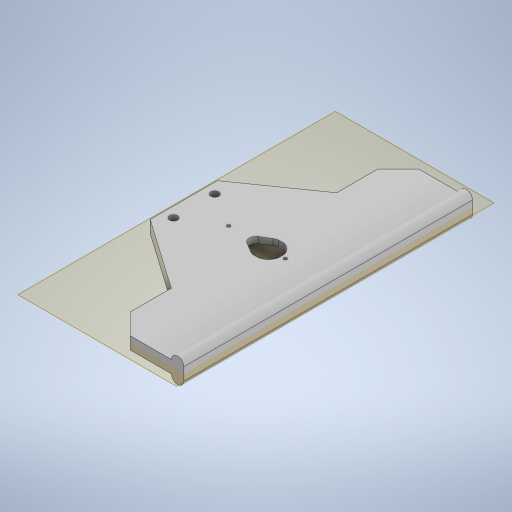
# Autodesk Inventor part: gripper_head 1
Saved by Autodesk Inventor 2023 (Build 270158000, 158)
## iProperties
Created: 2024-07-03
Part Number: gripper_head 1
Material: Generic
Document SubType Name: Modeling
Designer: Swoby
Density: 1 g/cm^3
Appearance: Default
Author: Swoby
Autodesk Inventor part; units mm, degrees
ref_plane "YZ Plane" through (0, 0, 0) normal (1, 0, 0) x (0, 1, 0)
ref_plane "XY Plane" through (0, 0, 0) normal (0, 0, 1) x (1, 0, 0)
sketch "Sketch1" plane through (0, 0, 0) normal (0, 0, 1) x (1, 0, 0)
  line L0 (-67, 3) -> (-67, -3)
  line L1 (-67, -3) -> (-3, -3)
  line L2 (-67, 3) -> (-3, 3)
  line L3 (0, -3) -> (0, 3) construction
  line L4 (3, -3) -> (3, 3)
  line L5 (-3, 3) -> (-3, -3)
  arc A0 (-3, -3) -> (3, -3) centre (0, -3) ccw
  arc A1 (3, 3) -> (-3, 3) centre (0, 3) ccw
  point P0 (0, 0)
  point P1 (-3, -3)
  dimension "d0" = 70
  dimension "d1" = 3
  dimension "d2" = 6
  dimension "d3" = 6
  constraints: 14 end point, 4 point on circle, 4 tangent, 2 centre point, 1 midpoint, 1 parallel, 1 perpendicular, 1 point on line, 1 vertical
  measures "d0" distance between parallel lines of L4 L0
  measures "d1" radius of A1
  measures "d2" distance between parallel lines of L1 L2
  measures "d3" distance of L3.start L3.end
extrude "Extrusion1" add sketch "Sketch1" along normal mid plane 140
sketch "Sketch2" plane through (-67, 3, 70) normal (0, 1, 0) x (1, 0, 0)
  line L0 (0, 0) -> (64, 0) projected
  line L1 (64, 0) -> (44, 0)
  line L2 (0, 140) -> (0, 0) projected
  line L3 (44, 0) -> (34, 10)
  line L4 (34, 10) -> (34, 29.9)
  line L5 (34, 29.9) -> (0, 53.7071)
  line L6 (0, 53.7071) -> (0, 86.2929)
  line L7 (0, 86.2929) -> (34, 110.1)
  line L8 (34, 110.1) -> (34, 130)
  line L9 (34, 130) -> (44, 140)
  line L10 (0, 140) -> (64, 140) projected
  line L11 (44, 140) -> (64, 140)
  line L12 (64, 140) -> (64, 0) projected
  point P0 (67, 70)
  dimension "d6" = 20
  dimension "d7" = 20
  dimension "d8" = 30
  dimension "d9" = 45
  dimension "d10" = 45
  dimension "d11" = 19.9
  dimension "d12" = 19.9
  dimension "d13" = 125
  dimension "d14" = 125
  constraints: 18 end point, 3 point on line, 2 collinear, 1 parallel, 1 vertical
  measures "d6" distance from line of L1.end L12
  measures "d7" distance from line of L12 L9.end
  measures "d8" distance between parallel lines of L12 L4
  measures "d9" angle of L0 L3
  measures "d10" angle of L10 L9
  measures "d11" distance of L3.end L4.end
  measures "d12" distance of L7.end L8.end
  measures "d13" angle of L5 L4
  measures "d14" angle of L7 L8
extrude "Extrusion2" cut sketch "Sketch2" against normal through all contours L2 L5 L4 L3 L0 | L2 L10 L9 L8 L7
sketch "Sketch3" plane through (-3, 3, 70) normal (0, 1, 0) x (1, 0, 0)
  circle A0 centre (-59, 80) radius 1.9
  circle A1 centre (-59, 60) radius 1.9
  line L0 (-64, 86.2929) -> (-64, 53.7071) projected
  line L1 (-59, 80) -> (-59, 60)
  point P0 (3, 70)
  point P1 (-64, 70)
  dimension "d17" = 3.8
  dimension "d18" = 3.8
  dimension "d19" = 20
  dimension "d20" = 10
  dimension "d21" = 5
  constraints: 2 centre point, 2 end point, 1 midpoint, 1 vertical
  measures "d17" diameter of A0
  measures "d18" diameter of A1
  measures "d19" distance of L1.end L1.start
  measures "d20" vertical distance of L1.start point (-64, 70)
  measures "d21" distance between parallel lines of L0 L1
extrude "Extrusion3" cut sketch "Sketch3" against normal through all
sketch "Sketch4" plane through (-3, 3, 70) normal (0, 1, 0) x (1, 0, 0)
  line L0 (-44.67, 64.05) -> (-12.45, 64.05)
  line L1 (-12.45, 64.05) -> (-12.45, 75.95)
  line L2 (-12.45, 75.95) -> (-44.67, 75.95)
  line L3 (-44.67, 75.95) -> (-44.67, 64.05)
  line L4 (-44.67, 64.05) -> (-12.45, 75.95) construction
  line L5 (-12.45, 64.05) -> (-44.67, 75.95) construction
  line L6 (6, 140) -> (6, 0) projected
  line L7 (6, 70) -> (-4, 70)
  line L8 (-40.17, 64.05) -> (-16.95, 64.05)
  line L9 (-16.95, 64.05) -> (-16.95, 75.95)
  line L10 (-16.95, 75.95) -> (-40.17, 75.95)
  line L11 (-40.17, 75.95) -> (-40.17, 64.05)
  line L12 (0, 140) -> (0, 0) projected
  line L13 (-44.87, 76.15) -> (-12.25, 76.15)
  line L14 (-12.25, 76.15) -> (-12.25, 63.85)
  line L15 (-12.25, 63.85) -> (-44.87, 63.85)
  line L16 (-44.87, 63.85) -> (-44.87, 76.15)
  line L17 (-47.37, 78.65) -> (-47.37, 61.35)
  line L18 (-9.75, 61.35) -> (-9.75, 78.65)
  circle A0 centre (-59, 80) radius 1.9 projected
  circle A1 centre (-59, 60) radius 1.9 projected
  line L19 (-47.37, 61.35) -> (-60.337, 61.35)
  line L20 (-57.663, 61.35) -> (-9.75, 61.35)
  line L21 (-9.75, 78.65) -> (-57.663, 78.65)
  line L22 (-60.337, 78.65) -> (-47.37, 78.65)
  circle A2 centre (-29, 70) radius 2.45
  point P0 (3, 70)
  point P1 (-28.56, 70)
  point P2 (-47.37, 78.65)
  point P3 (-47.37, 61.35)
  point P4 (-57.663, 61.35)
  point P5 (-57.663, 78.65)
  dimension "d24" = 32.22
  dimension "d25" = 11.9
  dimension "d26" = 4.5
  dimension "d27" = 4.5
  dimension "d30" = 0.2
  dimension "d34" = 2.5
  dimension "d35" = 2.5
  dimension "d36" = 2.5
  dimension "d37" = 2.5
  dimension "d51" = 29
  dimension "d52" = 12.05
  dimension "d53" = 4.9
  constraints: 42 end point, 11 parallel, 5 perpendicular, 5 point on line, 4 point on circle, 3 horizontal, 3 midpoint, 2 collinear, 1 centre point, 3 other
  measures "d24" distance of L1.end L2.end
  measures "d25" distance of L0.end L1.end
  measures "d26" distance between parallel lines of L3 L11
  measures "d27" distance between parallel lines of L1 L9
  measures "d30" distance between parallel lines of L2 L13
  measures "d34" distance between parallel lines of L17 L16
  measures "d35" distance between parallel lines of L18 L14
  measures "d36" distance between parallel lines of L13 L21
  measures "d37" distance between parallel lines of L20 L15
  measures "d51" distance from line of L12 A2.centre
  measures "d52" distance from line of L9 A2.centre
  measures "d53" diameter of A2
extrude "Extrusion4" add sketch "Sketch4" against normal blind 15 contours L3 L2 L11 L0 | L11 L2 L9 L0 | L9 L2 L1 L0 | L13 L14 L15 L16 | L21 L18 L20 L17 | A2
sketch "Sketch5" plane through (-3, -12, 70) normal (0, -1, 0) x (1, 0, 0)
  circle A0 centre (-59, -80) radius 1.9 projected
  circle A1 centre (-59, -60) radius 1.9 projected
  line L0 (-30, -110.1) -> (-64, -86.2929) projected
  line L1 (-64, -86.2929) -> (-64, -53.7071) projected
  line L2 (-64, -53.7071) -> (-30, -29.9) projected
  line L3 (-30, -29.9) -> (-30, -10) projected
  line L4 (-30, -10) -> (-20, 0) projected
  line L5 (0, 0) -> (-20, 0) projected
  line L6 (0, -140) -> (0, 0) projected
  line L7 (-20, -140) -> (0, -140) projected
  line L8 (-20, -140) -> (-30, -130) projected
  line L9 (-30, -130) -> (-30, -110.1) projected
  line L10 (-12.45, -75.95) -> (-44.67, -75.95) projected
  line L11 (-16.95, -64.05) -> (-16.95, -75.95) projected
  line L12 (-44.87, -76.15) -> (-12.25, -76.15) projected
  line L13 (-12.25, -76.15) -> (-12.25, -63.85) projected
  line L14 (-12.45, -64.05) -> (-12.45, -75.95) projected
  line L15 (-44.67, -64.05) -> (-12.45, -64.05) projected
  line L16 (-12.25, -63.85) -> (-44.87, -63.85) projected
  line L17 (-44.87, -63.85) -> (-44.87, -76.15) projected
  line L18 (-44.67, -75.95) -> (-44.67, -64.05) projected
  line L19 (-44.67, -64.05) -> (-12.45, -75.95) construction
  line L20 (-40.17, -75.95) -> (-40.17, -64.05) projected
  line L21 (-40.17, -75.95) -> (-40.17, -76.15)
  line L22 (-40.17, -64.05) -> (-40.17, -63.85)
  line L23 (-16.95, -76.15) -> (-16.95, -75.95)
  line L24 (-16.95, -64.05) -> (-16.95, -63.85)
  point P0 (3, -70)
  constraints: 8 end point, 7 point on line, 1 collinear
extrude "Extrusion5" cut sketch "Sketch5" against normal blind 7 contours L14 L15 L24 L16 L13 L12 L23 L10 | L10 L11 L15 L14 | L23 L12 L21 L10 | L10 L20 L15 L11 | L21 L12 L17 L16 L22 L15 L18 L10 | L10 L18 L15 L20 | L15 L22 L16 L24
sketch "Sketch6" plane through (-3, -5, 70) normal (0, -1, 0) x (1, 0, 0)
  line L0 (-16.95, -64.05) -> (-16.95, -75.95) construction
  line L1 (-12.45, -64.05) -> (-44.67, -75.95) construction
  line L2 (-40.17, -75.95) -> (-40.17, -64.05) construction
  line L3 (-12.25, -63.85) -> (-12.25, -76.15) projected
  line L4 (-44.87, -63.85) -> (-12.25, -63.85) projected
  line L5 (-44.87, -76.15) -> (-44.87, -63.85) projected
  line L6 (-12.25, -76.15) -> (-44.87, -76.15) projected
  line L7 (-16.95, -64.05) -> (-16.95, -63.85)
  line L8 (-44.87, -63.85) -> (-12.25, -63.85) projected
  line L9 (-16.95, -75.95) -> (-16.95, -76.15)
  line L10 (-40.17, -76.15) -> (-40.17, -75.95)
  line L11 (-40.17, -64.05) -> (-40.17, -63.85)
  line L12 (-40.32, -76.15) -> (-40.32, -63.85)
  line L13 (-16.8, -76.15) -> (-16.8, -63.85)
  line L14 (-40.32, -76.15) -> (-16.8, -76.15)
  line L15 (-16.8, -76.15) -> (-16.8, -63.85)
  line L16 (-16.8, -63.85) -> (-40.32, -63.85)
  line L17 (-40.32, -63.85) -> (-40.32, -76.15)
  point P0 (3, -70)
  dimension "d40" = 0.15
  dimension "d41" = 0.15
  constraints: 20 end point, 10 point on line, 4 parallel, 3 perpendicular, 1 horizontal
  measures "d40" distance between parallel lines of L2 L12
  measures "d41" distance between parallel lines of L13 L0
extrude "Extrusion6" cut sketch "Sketch6" against normal blind 5 contours L13 L6 L12 L4
sketch "Sketch7" plane through (-3, 0, 70) normal (0, -1, 0) x (1, 0, 0)
  line L0 (-16.8, -63.85) -> (-16.8, -76.15) projected
  line L1 (-16.8, -70) -> (-21, -70)
  circle A0 centre (-22.95, -70) radius 6.15 construction
  line L2 (-44.87, -63.85) -> (-12.25, -63.85) projected
  arc A1 (-24.3166, -63.85) -> (-24.3166, -76.15) centre (-22.95, -70) ccw
  circle A2 centre (-28.8, -70) radius 3 construction
  line L3 (-24.3166, -63.85) -> (-30.3313, -67.4202) construction
  line L4 (-30.3313, -72.5798) -> (-24.3166, -76.15) construction
  line L5 (-12.25, -76.15) -> (-44.87, -76.15) projected
  arc A3 (-21.5834, -63.85) -> (-24.3166, -63.85) centre (-22.95, -70) ccw construction
  arc A4 (-21.5834, -76.15) -> (-16.8, -71.3666) centre (-22.95, -70) ccw
  arc A5 (-24.3166, -76.15) -> (-21.5834, -76.15) centre (-22.95, -70) ccw construction
  arc A6 (-16.8, -71.3666) -> (-16.8, -68.6334) centre (-22.95, -70) ccw construction
  arc A7 (-16.8, -68.6334) -> (-21.5834, -63.85) centre (-22.95, -70) ccw
  line L6 (-26.1657, -64.5825) -> (-30.4916, -67.1503)
  arc A8 (-28.169, -66.7467) -> (-28.3286, -66.7197) centre (-28.8, -70) ccw
  arc A9 (-30.4916, -67.1503) -> (-30.4916, -72.8497) centre (-28.8, -70) ccw
  line L7 (-30.4916, -72.8497) -> (-26.1657, -75.4175)
  point P0 (3, -70)
  dimension "d44" = 0.15
  dimension "d45" = 6
  dimension "d46" = 12
  constraints: 22 point on circle, 10 end point, 9 centre point, 8 point on line, 5 tangent, 2 midpoint, 2 parallel, 1 horizontal, 1 perpendicular, 1 vertical, 3 other
  measures "d45" diameter of A2
  measures "d46" distance of A2.centre point (-16.8, -70)
extrude "Extrusion7" cut sketch "Sketch7" against normal through all contours L0 A4 L5 A1 L2 A7 | A1 L7 A9 L6
fillet "Fillet1" radius 2 4 edges at (-12.75, -7.5, -8.65) (-50.37, -7.5, -8.65) (-50.37, -7.5, 8.65) (-12.75, -7.5, 8.65)
sketch "Sketch9" plane through (-3, -5, 70) normal (0, -1, 0) x (1, 0, 0)
  circle A0 centre (-14.81, -70) radius 0.8
  line L0 (3, -70) -> (-41.3866, -70) construction
  line L1 (-40.32, -76.15) -> (-40.32, -63.85) projected
  line L2 (6, -140) -> (6, 0) projected
  circle A1 centre (-42.31, -70) radius 0.8
  dimension "d64" = 1.6
  dimension "d65" = 20.81
  dimension "d66" = 1.6
  dimension "d67" = 27.5
  constraints: 2 centre point, 2 end point, 2 point on line, 1 perpendicular
  measures "d64" diameter of A0
  measures "d65" distance from line of L2 A0.centre
  measures "d66" diameter of A1
  measures "d67" distance of A0.centre A1.centre
extrude "Extrusion9" cut sketch "Sketch9" against normal blind 8
sketch "Sketch10" plane through (-3, -5, 70) normal (0, -1, 0) x (1, 0, 0)
  circle A0 centre (-14.81, -70) radius 0.8 projected
  circle A1 centre (-42.31, -70) radius 0.8 projected
  line L0 (-12.4678, -70) -> (-46, -70)
  line L1 (-44.87, -63.85) -> (-12.25, -63.85) projected
  line L2 (-12.25, -63.85) -> (-12.25, -76.15) projected
  line L3 (-12.25, -76.15) -> (-44.87, -76.15) projected
  line L4 (-44.87, -76.15) -> (-44.87, -63.85) projected
  arc A2 (-9.75, -63.35) -> (-11.75, -61.35) centre (-11.75, -63.35) ccw projected
  line L5 (-11.75, -61.35) -> (-45.37, -61.35) projected
  arc A3 (-45.37, -61.35) -> (-47.37, -63.35) centre (-45.37, -63.35) ccw projected
  line L6 (-47.37, -63.35) -> (-47.37, -76.65) projected
  arc A4 (-47.37, -76.65) -> (-45.37, -78.65) centre (-45.37, -76.65) ccw projected
  line L7 (-45.37, -78.65) -> (-11.75, -78.65) projected
  arc A5 (-11.75, -78.65) -> (-9.75, -76.65) centre (-11.75, -76.65) ccw projected
  line L8 (-9.75, -76.65) -> (-9.75, -63.35) projected
  line L9 (-10.75, -63.35) -> (-10.75, -76.65)
  line L10 (-46.37, -64) -> (-46.37, -74.4084)
  circle A6 centre (-43.87, -70) radius 2.5
  circle A7 centre (-13.25, -70) radius 2.5
  point P0 (3, -70)
  point P1 (-44.87, -67.7087)
  point P2 (-44.87, -72.2913)
  point P3 (-12.25, -67.7087)
  point P4 (-12.25, -72.2913)
  dimension "d70" = 1
  dimension "d71" = 1
  dimension "d72" = 5
  dimension "d73" = 5
  constraints: 6 end point, 3 point on line, 2 centre point, 2 tangent, 2 vertical, 1 horizontal
  measures "d70" distance between parallel lines of L9 L8
  measures "d71" distance between parallel lines of L6 L10
  measures "d72" diameter of A6
  measures "d73" diameter of A7
extrude "Extrusion10" cut sketch "Sketch10" along normal through all contours L4 A6 | A7 L2 picked at (-11.5834, -70.097)
chamfer "Chamfer1" distance 1 angle 45 4 edges at (-15.25, -8.5, -2.2913) (-15.25, -8.5, 2.2913) (-47.87, -8.5, -2.2913) (-47.87, -8.5, 2.2913)
equation "\"d7\" = d6"
equation "\"d10\" = d9"
equation "\"d12\" = d11"
equation "\"d14\" = d13"
equation "\"d17\" = d18"
equation "\"d27\" = d26"
equation "\"d34\" = d36"
equation "\"d35\" = d36"
equation "\"d37\" = d36"
body "Solid1"
